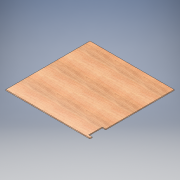
# Autodesk Inventor part: КВ33.044.005 - Крышка блока управления
Saved by Autodesk Inventor 2019 (Build 230136000, 136)
## iProperties
Created: 2019-08-11
Part Number: КВ33.044.005 - Крышка блока управления
Material: Дерево (береза)
Document SubType Name: Modeling
Designer: Петров Иван
Density: 0.55 g/cm^3
Appearance: Береза — натуральный — полированный
Author: Петров Иван
Autodesk Inventor part; units mm, degrees
ref_plane "YZ Plane" through (0, 0, 0) normal (1, 0, 0) x (0, 1, 0)
ref_plane "XZ Plane" through (0, 0, 0) normal (0, 1, 0) x (-1, 0, 0)
ref_plane "XY Plane" through (0, 0, 0) normal (0, 0, 1) x (1, 0, 0)
sketch "Эскиз1" plane through (0, 0, 0) normal (0, 1, 0) x (-1, 0, 0)
  line L0 (-370, 370) -> (370, 370)
  line L1 (370, 370) -> (370, -370)
  line L2 (370, -370) -> (-370, -370)
  line L3 (-370, -370) -> (-370, 370)
  line L4 (-370, 370) -> (370, -370) construction
  line L5 (370, 370) -> (-370, -370) construction
  point P0 (0, 0)
  dimension "d0" = 740
  dimension "d1" = 740
  constraints: 12 end point, 2 midpoint, 2 parallel, 1 horizontal, 1 perpendicular
  measures "d0" distance of L1.end L2.end
  measures "d1" distance of L0.end L1.end
extrude "Выдавливание1" add sketch "Эскиз1" along normal blind 8
sketch "Эскиз2" plane through (0, 8, 0) normal (0, 1, 0) x (1, 0, 0)
  line L0 (370, -370) -> (370, 370) projected
  line L1 (370, -352.0422) -> (340, -352.0422)
  line L2 (340, -352.0422) -> (340, -232.0422)
  line L3 (340, -232.0422) -> (370, -232.0422)
  line L4 (370, -232.0422) -> (370, -352.0422)
  point P0 (0, 0)
  dimension "d4" = 30
  dimension "d5" = 120
  constraints: 8 end point, 2 parallel, 1 horizontal, 1 perpendicular, 1 point on line
  measures "d4" distance of L2.end L3.end
  measures "d5" distance of L1.end L2.end
extrude "Выдавливание2" cut sketch "Эскиз2" against normal blind 8
